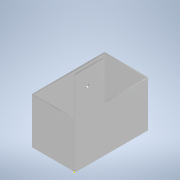
# Autodesk Inventor part: box
Saved by Autodesk Inventor 2021 (Build 250183000, 183)
## iProperties
Created: 2021-06-22
Part Number: box
Material: Aluminum 6061
Document SubType Name: Modeling
Designer: Watchdog
Density: 2.7 g/cm^3
Appearance: Aluminum - Flat
Mass: 1563.93 g
Surface Area: 3807.83 cm^2
Volume: 579.233 cm^3
Author: Watchdog
Autodesk Inventor part; units mm, degrees
ref_plane "YZ Plane" through (0, 0, 0) normal (1, 0, 0) x (0, 1, 0)
ref_plane "XZ Plane" through (0, 0, 0) normal (0, 1, 0) x (-1, 0, 0)
ref_plane "XY Plane" through (0, 0, 0) normal (0, 0, 1) x (1, 0, 0)
sketch "Sketch1" plane through (0, 0, 0) normal (0, 1, 0) x (-1, 0, 0)
  line L0 (0, -188) -> (-113, -188)
  line L1 (-113, -188) -> (-113, 0)
  line L2 (-113, 0) -> (0, 0)
  line L3 (0, 0) -> (0, -188)
  dimension "d26" = 188
  dimension "d27" = 113
  constraints: 8 end point, 2 parallel, 1 coincident, 1 horizontal, 1 perpendicular
  measures "d26" distance between parallel lines of L2 L0
  measures "d27" distance of L0.start L0.end
extrude "base" add sketch "Sketch1" along normal blind 3
sketch "Sketch7" plane through (0, 3, 0) normal (0, 1, 0) x (1, 0, 0)
  line L0 (113, 188) -> (0, 188) projected
  line L1 (0, 0) -> (113, 0) projected
  line L2 (113, 0) -> (113, 188) projected
  line L3 (113, 188) -> (0, 188) projected
  line L4 (0, 188) -> (0, 0) projected
  line L5 (3, 3) -> (110, 3)
  line L6 (110, 3) -> (110, 185)
  line L7 (110, 185) -> (3, 185)
  line L8 (3, 185) -> (3, 3)
  dimension "d29" = 3
  constraints: 8 end point, 3 other
  measures "d29" distance between parallel lines of L4 L8
extrude "walls" add sketch "Sketch7" along normal blind 115
sketch "Sketch13" plane through (3, 3, -185) normal (0, 0, 1) x (1, 0, 0)
  line L0 (107, 0) -> (0, 0) projected
  line L1 (65, 0) -> (68, 0)
  line L2 (68, 0) -> (68, 65)
  line L3 (68, 65) -> (65, 65)
  line L4 (65, 65) -> (65, 0)
  line L5 (0, 0) -> (0, 115) projected
  point P0 (-3, -3)
  point P1 (68, 0)
  dimension "d93" = 3
  dimension "d94" = 65
  dimension "d150" = 65
  constraints: 8 end point, 2 parallel, 1 horizontal, 1 perpendicular, 1 point on line
  measures "d93" distance of L3.end L2.end
  measures "d94" distance of L1.end L2.end
  measures "d150" distance between parallel lines of L5 L4
extrude "Extrusion8" add sketch "Sketch13" along normal blind 54
sketch "Sketch14" plane through (68, 3, -185) normal (-1, 0, 0) x (0, 0, 1)
  circle A0 centre (30, 36) radius 18
  line L0 (30, 36) -> (14.4115, 27)
  line L1 (30, 36) -> (30, 54)
  line L2 (30, 36) -> (45.5885, 27)
  line L3 (54, 0) -> (0, 0) projected
  line L4 (54, 65) -> (54, 0) projected
  line L5 (0, 0) -> (0, 115) projected
  point P0 (185, -3)
  dimension "d98" = 36
  dimension "d99" = 120
  dimension "d100" = 120
  dimension "d101" = 36
  dimension "d114" = 30
  constraints: 6 end point, 3 coincident, 3 point on circle, 1 centre point, 1 vertical
  measures "d98" diameter of A0
  measures "d99" angle of L1 L0
  measures "d100" angle of L1 L2
  measures "d101" distance from line of L3 L0.start
  measures "d114" distance from line of L5 L0.start
hole "Hole4" at (68, 30, -170.5885) at (68, 57, -155) at (68, 30, -139.4115) direction (1, 0, 0) diameter 6 depth 3 tip angle 118
fillet "Fillet2" radius 1 6 edges at (69.5, 68, -185) (68, 35.5, -185) (71, 35.5, -185) (71, 3, -158) (68, 3, -158) (69.5, 3, -131)
sketch "Sketch15" plane through (68, 4, -131) normal (-1, 0, 0) x (0, 0, 1)
  circle A0 centre (-24, 36) radius 12.5
  line L0 (0, 0) -> (-53, 0) projected
  line L1 (-54, 65) -> (-54, -1) projected
  point P0 (131, -4)
  dimension "d111" = 25
  dimension "d115" = 36
  dimension "d116" = 30
  constraints: 1 centre point
  measures "d111" diameter of A0
  measures "d115" distance from line of L0 A0.centre
  measures "d116" distance from line of L1 A0.centre
extrude "Extrusion9" cut sketch "Sketch15" against normal up to surface (3 mm away)
fillet "Fillet3" radius 30 1 edges at (69.5, 68, -131)
sketch "Sketch17" plane through (0, 118, 0) normal (0, 1, 0) x (1, 0, 0)
  line L0 (0, 188) -> (113, 188)
  line L1 (113, 188) -> (113, 0)
  line L2 (113, 0) -> (0, 0)
  line L3 (0, 0) -> (0, 188)
  point P0 (0, 0)
  constraints: 8 end point, 2 parallel, 1 horizontal, 1 perpendicular
extrude "Extrusion11" [suppressed]
chamfer "Chamfer4" distance 1.5 angle 45 7 edges at (0, 59, -188) (113, 59, -188) (0, 59, 0) (0, 0, -94) (56.5, 0, -188) (56.5, 0, 0) (113, 0, -94)
sketch "Sketch19" plane through (110, 3, -185) normal (-1, 0, 0) x (0, 0, 1)
  point P0 (185, -3)
sketch "Sketch20" plane through (0, 118, 0) normal (0, 1, 0) x (1, 0, 0)
  line L0 (110, 185) -> (110, 3) projected
  line L1 (113, 0) -> (110, 0)
  line L2 (110, 0) -> (110, 75)
  line L3 (110, 75) -> (113, 75)
  line L4 (113, 75) -> (113, 0)
  point P0 (0, 0)
  dimension "d151" = 75
  constraints: 8 end point, 2 parallel, 1 horizontal, 1 perpendicular, 1 point on line
  measures "d151" distance between parallel lines of L1 L3
extrude "Extrusion12" add sketch "Sketch20" along normal blind 100
sketch "Sketch21" plane through (113, 1.5, -186.5) normal (1, 0, 0) x (0, 0, -1)
  line L0 (-186.5, 216.5) -> (-111.5, 216.5) projected
  line L1 (-186.5, 0) -> (-186.5, 216.5) projected
  point P0 (-186.5, -1.5)
  point P1 (-156.5, 178.5)
  dimension "d154" = 38
  dimension "d155" = 30
  measures "d154" distance from line of L0 point (-156.5, 178.5)
  measures "d155" distance from line of L1 point (-156.5, 178.5)
hole "Hole6" at (113, 180, -30) direction (-1, 0, 0) diameter 12 end through all
equation "\"d0\" = t"
equation "\"d29\" = t"
equation "\"d93\" = t"
equation "\"d128\" = t"
equation "\"t\" = 3"
equation "\"pd\" = 28"
equation "\"dmotorpattern\" = 36"
equation "\"d72\" = 36"
equation "\"d73\" = 28"
body "Solid1"
